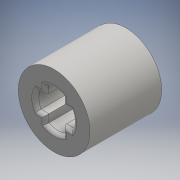
# Autodesk Inventor part: dif-coupler
Saved by Autodesk Inventor 2016 (Build 200138000, 138)
## iProperties
Created: 2024-02-03
Part Number: dif-coupler
Material: Generic
Document SubType Name: Modeling
Designer: Dell
Density: 1 g/cm^3
Appearance: Default
Author: Dell
Autodesk Inventor part; units mm, degrees
ref_plane "YZ Plane" through (0, 0, 0) normal (1, 0, 0) x (0, 1, 0)
ref_plane "XZ Plane" through (0, 0, 0) normal (0, 1, 0) x (-1, 0, 0)
ref_plane "XY Plane" through (0, 0, 0) normal (0, 0, 1) x (1, 0, 0)
sketch "Sketch1" plane through (0, 0, 0) normal (0, 1, 0) x (-1, 0, 0)
  line L0 (2.2361, -2) -> (-2.2361, -2)
  line L1 (2.2361, 2) -> (-2.2361, 2)
  arc A0 (2.2361, -2) -> (2.2361, 2) centre (0, 0) ccw
  arc A1 (-2.2361, 2) -> (-2.2361, -2) centre (0, 0) ccw
  circle A2 centre (0, 0) radius 5
  dimension "d1" = 2
  dimension "d2" = 2
  dimension "d3" = 10
  dimension "d20" = 3
  dimension "d21" = 3
  constraints: 4 end point, 4 point on circle, 3 centre point, 2 coincident, 2 horizontal
  measures "d1" distance from line of point (0, 0) L0
  measures "d2" distance from line of point (0, 0) L1
  measures "d3" diameter of A2
  measures "d20" radius of A0
  measures "d21" radius of A1
extrude "Extrusion1" add sketch "Sketch1" along normal blind 5
sketch "Sketch2" plane through (0, 0, 0) normal (0, -1, 0) x (1, 0, 0)
  circle A0 centre (0, 0) radius 5
  dimension "d19" = 10
  constraints: 1 centre point, 1 coincident
  measures "d19" diameter of A0
extrude "Extrusion2" add sketch "Sketch2" along normal blind 5
sketch "Sketch3" plane through (0, -5, 0) normal (0, -1, 0) x (1, 0, 0)
  circle A0 centre (0, 0) radius 2.625
  line L0 (1.2228, 2.3228) -> (1.2228, 1.2228)
  line L1 (1.2228, -1.2228) -> (1.2228, -2.3228)
  line L2 (2.3228, -1.2228) -> (1.2228, -1.2228)
  line L3 (-1.2228, -1.2228) -> (-2.3228, -1.2228)
  line L4 (2.3228, 1.2228) -> (1.2228, 1.2228)
  line L5 (-1.2228, 1.2228) -> (-2.3228, 1.2228)
  line L6 (-1.2228, 2.3228) -> (-1.2228, 1.2228)
  line L7 (-1.2228, -1.2228) -> (-1.2228, -2.3228)
  dimension "d10" = 5.25
  dimension "d22" = 1.1
  dimension "d23" = 1.1
  dimension "d24" = 1.1
  dimension "d25" = 1.1
  dimension "d26" = 1.1
  dimension "d27" = 1.1
  dimension "d28" = 1.1
  dimension "d29" = 1.1
  constraints: 16 end point, 4 horizontal, 4 vertical, 1 coincident, 10 other
  measures "d22" distance of L5.start L5.end
  measures "d23" distance of L6.start L5.start
  measures "d24" distance of L3.start L3.end
  measures "d25" distance of L3.start L7.end
  measures "d26" distance of L4.start L0.end
  measures "d27" distance of L0.start L0.end
  measures "d28" distance of L2.start L1.start
  measures "d29" distance of L1.start L1.end
extrude "Extrusion3" cut sketch "Sketch3" against normal blind 5 contours A0 L2 L1 L7 L3 L5 L6 L0 L4
fillet "Fillet2" radius 0.5 12 edges at (2.625, -5, 0) (1.7728, -5, 1.2228) (1.2228, -5, 1.7728) (0, -5, 2.625) (-1.2228, -5, 1.7728) (-2.625, -5, 0) (-1.7728, -5, 1.2228) (-1.7728, -5, -1.2228) (-1.2228, -5, -1.7728) (0, -5, -2.625) (1.7728, -5, -1.2228) (1.2228, -5, -1.7728)
equation "\"d23\" = d22"
equation "\"d24\" = d22"
equation "\"d25\" = d22"
equation "\"d26\" = d22"
equation "\"d27\" = d22"
equation "\"d28\" = d22"
equation "\"d29\" = d22"
body "Solid1"
